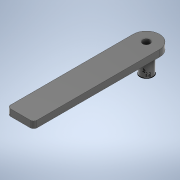
# Autodesk Inventor part: CC-topHand
Saved by Autodesk Inventor 2020 (Build 240168000, 168)
## iProperties
Created: 2019-07-03
Part Number: CC-topHand
Material: ABS Plastic
Document SubType Name: Modeling
Designer: andwh
Density: 1.06 g/cm^3
Appearance: Smooth - Black
Author: andwh
Autodesk Inventor part; units mm, degrees
ref_plane "YZ Plane" through (0, 0, 0) normal (1, 0, 0) x (0, 1, 0)
ref_plane "XZ Plane" through (0, 0, 0) normal (0, 1, 0) x (-1, 0, 0)
ref_plane "XY Plane" through (0, 0, 0) normal (0, 0, 1) x (1, 0, 0)
sketch "Sketch1" plane through (0, 0, 0) normal (0, 1, 0) x (-1, 0, 0)
  circle A0 centre (0, 0) radius 1.9
  circle A1 centre (0, 0) radius 1.1
  dimension "d0" = 3.8
  dimension "d1" = 2.2
  constraints: 2 centre point, 2 coincident
  measures "d0" diameter of A0
  measures "d1" diameter of A1
extrude "Extrusion1" add sketch "Sketch1" along normal blind 6.2
sketch "Sketch2" plane through (0, 6.2, 0) normal (0, 1, 0) x (1, 0, 0)
  line L0 (0, 0) -> (0, -38.1) construction
  line L1 (-4, 0) -> (-4, -38.1)
  line L2 (4, -38.1) -> (4, 0)
  arc A0 (4, 0) -> (-4, 0) centre (0, 0) ccw
  line L3 (4, -38.1) -> (-4, -38.1)
  circle A1 centre (0, 0) radius 1.1 projected
  point P0 (0, -19.05)
  dimension "d6" = 4
  dimension "d7" = 38.1
  constraints: 10 end point, 2 midpoint, 2 point on circle, 2 tangent, 1 centre point, 1 horizontal, 1 parallel, 1 vertical
  measures "d6" radius of A0
  measures "d7" distance of L0.start L0.end
extrude "Extrusion2" add sketch "Sketch2" along normal blind 2
sketch "Sketch3" plane through (0, 6.2, 0) normal (0, -1, 0) x (1, 0, 0)
  circle A0 centre (0, 30.48) radius 1.5
  circle A1 centre (0, 0) radius 1.9 projected
  dimension "d11" = 3
  dimension "d12" = 30.48
  constraints: 1 centre point, 1 vertical alignment
  measures "d11" diameter of A0
  measures "d12" distance of A0.centre A1.centre
extrude "Extrusion3" cut sketch "Sketch3" against normal blind 1 contours A0
fillet "Fillet1" radius 1 2 edges at (-4, 7.2, 38.1) (4, 7.2, 38.1)
body "Solid1"
